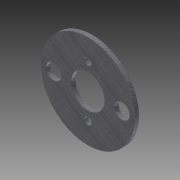
# Autodesk Inventor part: Spring Ring BD drill motor mount
Saved by Autodesk Inventor 2012 (Build 160160000, 160)
## iProperties
Created: 2012-06-30
Part Number: Spring Ring BD drill motor mount
Material: Default
Document SubType Name: Modeling
Designer: Bruce
Density: 1 g/cm^3
Author: Bruce
Autodesk Inventor part; units mm, degrees
ref_plane "YZ Plane" through (0, 0, 0) normal (1, 0, 0) x (0, 1, 0)
ref_plane "XZ Plane" through (0, 0, 0) normal (0, 1, 0) x (-1, 0, 0)
ref_plane "XY Plane" through (0, 0, 0) normal (0, 0, 1) x (1, 0, 0)
sketch "Sketch1" plane through (0, 0, 0) normal (0, 0, 1) x (1, 0, 0)
  circle A0 centre (0, 0) radius 21.7805
  circle A1 centre (0, 0) radius 7.7788
  circle A2 centre (0, 0) radius 11.9888 construction
  circle A3 centre (-15.875, 0) radius 3.556
  circle A4 centre (15.875, 0) radius 3.556
  point P0 (0, 11.9888)
  point P1 (0, -11.9888)
  point P2 (0, 11.9888)
  point P3 (0, -11.9888)
  dimension "d0" = 43.561
  dimension "d1" = 15.5575
  dimension "d2" = 23.9776
  dimension "d3" = 7.112
  dimension "d4" = 7.112
  dimension "d5" = 31.75
  dimension "d6" = 15.875
  constraints: 5 centre point, 5 coincident, 2 horizontal alignment, 2 point on circle, 2 vertical alignment
  measures "d0" diameter of A0
  measures "d1" diameter of A1
  measures "d2" diameter of A2
  measures "d3" diameter of A3
  measures "d4" diameter of A4
  measures "d5" distance of A4.centre A3.centre
  measures "d6" distance of point (0, 0) A3.centre
extrude "Extrusion1" add sketch "Sketch1" against normal blind 1.9812
hole "Hole1" at (0, 11.9888, 0) at (0, -11.9888, 0) direction (0, 0, -1) diameter 3.302 end through all
equation "\"d4\" = d3"
equation "\"d6\" = 0.5 * d5"
body "Solid1"
